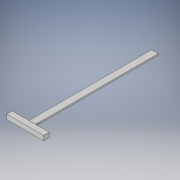
# Autodesk Inventor part: hopper stand
Saved by Autodesk Inventor 2019 (Build 230136000, 136)
## iProperties
Created: 2020-02-12
Part Number: hopper stand
Material: Generic
Document SubType Name: Modeling
Designer: ASUS
Density: 1 g/cm^3
Appearance: Default
Author: ASUS
Autodesk Inventor part; units mm, degrees
ref_plane "YZ Plane" through (0, 0, 0) normal (1, 0, 0) x (0, 1, 0)
ref_plane "XZ Plane" through (0, 0, 0) normal (0, 1, 0) x (-1, 0, 0)
ref_plane "XY Plane" through (0, 0, 0) normal (0, 0, 1) x (1, 0, 0)
sketch "Sketch1" plane through (0, 0, 0) normal (0, 1, 0) x (-1, 0, 0)
  line L0 (25.4, -475) -> (-25.4, -475)
  line L1 (-25.4, -475) -> (-25.4, 475)
  line L2 (-25.4, 475) -> (25.4, 475)
  line L3 (25.4, 475) -> (25.4, -475)
  line L4 (25.4, -475) -> (-25.4, 475) construction
  line L5 (-25.4, -475) -> (25.4, 475) construction
  point P0 (0, 0)
  dimension "d0" = 50.8
  dimension "d1" = 950
  constraints: 12 end point, 2 midpoint, 2 parallel, 1 horizontal, 1 perpendicular
  measures "d0" distance of L1.end L2.end
  measures "d1" distance of L0.end L1.end
extrude "Extrusion1" add sketch "Sketch1" along normal blind 12
sketch "Sketch2" plane through (0, 12, 0) normal (0, 1, 0) x (1, 0, 0)
  line L0 (142.2351, -433.1412) -> (-142.2351, -433.1412)
  line L1 (-142.2351, -433.1412) -> (-142.2351, -475.6186)
  line L2 (-142.2351, -475.6186) -> (142.2351, -475.6186)
  line L3 (142.2351, -475.6186) -> (142.2351, -433.1412)
  line L4 (142.2351, -433.1412) -> (-142.2351, -475.6186) construction
  line L5 (-142.2351, -433.1412) -> (142.2351, -475.6186) construction
  point P0 (0, 0)
  point P1 (0, -454.3799)
  constraints: 12 end point, 2 midpoint, 2 parallel, 1 horizontal, 1 perpendicular
extrude "Extrusion2" add sketch "Sketch2" along normal blind 12 and the other way blind 24
sketch "Sketch3" plane through (0, 12, 0) normal (0, 1, 0) x (1, 0, 0)
  line L0 (-638.112, 621.7865) -> (344.254, 621.7865)
  line L1 (344.254, 621.7865) -> (344.254, 342.1246)
  line L2 (344.254, 342.1246) -> (-638.112, 342.1246)
  line L3 (-638.112, 342.1246) -> (-638.112, 621.7865)
  line L4 (-638.112, 621.7865) -> (344.254, 342.1246) construction
  line L5 (344.254, 621.7865) -> (-638.112, 342.1246) construction
  point P0 (0, 0)
  point P1 (-146.929, 481.9555)
  constraints: 12 end point, 2 midpoint, 2 parallel, 1 horizontal, 1 perpendicular
extrude "Extrusion3" cut sketch "Sketch3" against normal blind 304.8 and the other way blind 152.4
sketch "Sketch4" plane through (0, 12, 0) normal (0, 1, 0) x (1, 0, 0)
  line L0 (-80.2076, 578.4886) -> (80.2076, 578.4886)
  line L1 (80.2076, 578.4886) -> (80.2076, 185.2583)
  line L2 (80.2076, 185.2583) -> (-80.2076, 185.2583)
  line L3 (-80.2076, 185.2583) -> (-80.2076, 578.4886)
  line L4 (-80.2076, 578.4886) -> (80.2076, 185.2583) construction
  line L5 (80.2076, 578.4886) -> (-80.2076, 185.2583) construction
  point P0 (0, 0)
  point P1 (0, 381.8735)
  constraints: 12 end point, 2 midpoint, 2 parallel, 1 horizontal, 1 perpendicular
extrude "Extrusion4" cut sketch "Sketch4" against normal blind 304.8
sketch "Sketch5" plane through (0, 0, 0) normal (0, 1, 0) x (-1, 0, 0)
  line L0 (-25.4, 475.4333) -> (25.4, 475.4333)
  line L1 (25.4, 475.4333) -> (25.4, -524.5667)
  line L2 (25.4, -524.5667) -> (-25.4, -524.5667)
  line L3 (-25.4, -524.5667) -> (-25.4, 475.4333)
  point P0 (0, 0)
  dimension "d14" = 50.8
  dimension "d15" = 1000
  constraints: 8 end point, 2 parallel, 1 horizontal, 1 perpendicular
  measures "d14" distance of L1.end L2.end
  measures "d15" distance of L0.end L1.end
extrude "Extrusion5" add sketch "Sketch5" along normal blind 12
sketch "Sketch6" plane through (0, 0, 0) normal (0, 1, 0) x (-1, 0, 0)
  point P0 (0, 0)
body "Solid1"
